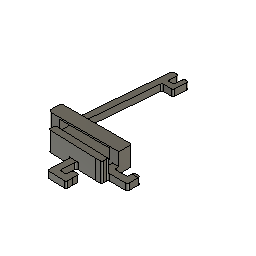
Keychain holder (Autodesk Fusion 360 design; units mm, degrees)
part number: 2026-04-03-17-33-08-056
Autodesk Fusion 360 part; units mm, degrees
note: some values were not read from the file. Chosen so that the rebuilt part matches the saved one: which bodies a step acts on.
sketch "Sketch1" plane through (0, 0, 0) normal (0, 0, 1) x (1, 0, 0)
  line L0 (0, 0) -> (0, 16.9)
  line L1 (0, 0) -> (-72.4203, 2.529)
  line L2 (0, 0) -> (75, 0) construction
  line L3 (0, 16.9) -> (-95, 16.9)
  line L4 (-100, 21.9) -> (-100, 34.4)
  line L5 (7.5, -10) -> (0, -10)
  line L6 (-75.0071, 0.0825) -> (-75.1109, -4.9108)
  line L7 (-89.5544, 39.1821) -> (-76.8804, 184.0471)
  line L8 (-79.7541, 36.9) -> (-9.7541, 36.9) construction
  line L9 (-74.3899, 186.3292) -> (-69.409, 186.3292)
  line L10 (-65.353, 170.3212) -> (-60.769, 170.3212)
  line L11 (-58.2785, 172.6033) -> (-57.3697, 182.9908)
  line L12 (-54.8792, 185.2729) -> (-52.7283, 185.2729)
  line L13 (-50.2378, 182.555) -> (-51.7942, 164.7646)
  line L14 (-54.2847, 162.4825) -> (-66.4762, 162.4825)
  line L15 (12.5, 10) -> (27.5, 10)
  line L16 (30, 12.5) -> (30, 17.5)
  line L17 (32.5, 20) -> (37.5, 20)
  line L18 (40, 17.5) -> (40, 2.5)
  line L19 (37.5, 0) -> (12.5, 0)
  line L20 (-30.1175, -11.4498) -> (-30.8155, -31.4376)
  line L21 (-28.4043, -34.0233) -> (-23.4057, -34.1979)
  line L22 (-10.9149, -34.6341) -> (-10.9149, -42.0453)
  line L23 (-13.5022, -44.5437) -> (-38.3982, -43.6743)
  line L24 (-40.8094, -41.0886) -> (-39.7626, -11.113)
  line L25 (-10.9149, -34.6341) -> (-10.6563, -27.2274)
  line L26 (-13.1548, -24.6402) -> (-18.1532, -24.6402)
  line L27 (-20.6517, -27.0513) -> (-20.8201, -31.7882)
  line L28 (-97.5, 36.9) -> (-92.0449, 36.9)
  line L29 (-77.0258, 36.9) -> (7.5, 36.9)
  line L30 (-66.9185, 183.6113) -> (-67.8435, 173.0391)
  line L31 (-68.9667, 160.2004) -> (-79.5163, 39.6179)
  line L32 (10, 34.4) -> (10, 12.5)
  line L33 (10, -2.5) -> (10, -7.5)
  line L34 (0, -10) -> (-27.5318, -9.0386)
  line L35 (-42.1739, -8.5273) -> (-72.6987, -7.4613)
  arc A0 (-74.3899, 186.3292) -> (-76.8804, 184.0471) centre (-74.3899, 183.8292) ccw
  arc A1 (-66.9185, 183.6113) -> (-69.409, 186.3292) centre (-69.409, 183.8292) ccw
  arc A2 (-50.2378, 182.555) -> (-52.7283, 185.2729) centre (-52.7283, 182.7729) ccw
  arc A3 (-54.8792, 185.2729) -> (-57.3697, 182.9908) centre (-54.8792, 182.7729) ccw
  arc A4 (-60.769, 170.3212) -> (-58.2785, 172.6033) centre (-60.769, 172.8212) ccw
  arc A5 (-67.8435, 173.0391) -> (-65.353, 170.3212) centre (-65.353, 172.8212) ccw
  arc A6 (-54.2847, 162.4825) -> (-51.7942, 164.7646) centre (-54.2847, 164.9825) ccw
  arc A7 (-66.4762, 162.4825) -> (-68.9667, 160.2004) centre (-66.4762, 159.9825) ccw
  arc A8 (-92.0449, 36.9) -> (-89.5544, 39.1821) centre (-92.0449, 39.4) ccw
  arc A9 (-79.5163, 39.6179) -> (-77.0258, 36.9) centre (-77.0258, 39.4) ccw
  arc A10 (10, 34.4) -> (7.5, 36.9) centre (7.5, 34.4) ccw
  arc A11 (10, 12.5) -> (12.5, 10) centre (12.5, 12.5) ccw
  arc A12 (27.5, 10) -> (30, 12.5) centre (27.5, 12.5) ccw
  arc A13 (32.5, 20) -> (30, 17.5) centre (32.5, 17.5) ccw
  arc A14 (40, 17.5) -> (37.5, 20) centre (37.5, 17.5) ccw
  arc A15 (37.5, 0) -> (40, 2.5) centre (37.5, 2.5) ccw
  arc A16 (12.5, 0) -> (10, -2.5) centre (12.5, -2.5) ccw
  arc A17 (7.5, -10) -> (10, -7.5) centre (7.5, -7.5) ccw
  arc A18 (-27.5318, -9.0386) -> (-30.1175, -11.4498) centre (-27.619, -11.537) ccw
  arc A19 (-30.8155, -31.4376) -> (-28.4043, -34.0233) centre (-28.317, -31.5249) ccw
  arc A20 (-23.4057, -34.1979) -> (-20.8201, -31.7882) centre (-23.3185, -31.6994) ccw
  arc A21 (-18.1532, -24.6402) -> (-20.6517, -27.0513) centre (-18.1532, -27.1402) ccw
  arc A22 (-10.6563, -27.2274) -> (-13.1548, -24.6402) centre (-13.1548, -27.1402) ccw
  arc A23 (-13.5022, -44.5437) -> (-10.9149, -42.0453) centre (-13.4149, -42.0453) ccw
  arc A24 (-40.8094, -41.0886) -> (-38.3982, -43.6743) centre (-38.3109, -41.1759) ccw
  arc A25 (-39.7626, -11.113) -> (-42.1739, -8.5273) centre (-42.2611, -11.0257) ccw
  arc A26 (-75.1109, -4.9108) -> (-72.6987, -7.4613) centre (-72.6115, -4.9628) ccw
  arc A27 (-72.4203, 2.529) -> (-75.0071, 0.0825) centre (-72.5076, 0.0305) ccw
  arc A28 (-97.5, 36.9) -> (-100, 34.4) centre (-97.5, 34.4) ccw
  arc A29 (-100, 21.9) -> (-95, 16.9) centre (-95, 21.9) ccw
  point P0 (-74.9543, 2.6175)
  point P1 (-100, 16.9)
  point P2 (-100, 36.9)
  point P3 (-89.7541, 36.9)
  point P4 (-76.6807, 186.3292)
  point P5 (30, 20)
  point P6 (40, 20)
  point P7 (-30.0303, -8.9513)
  point P8 (-30.9027, -33.9361)
  point P9 (-10.9149, -44.6341)
  point P10 (-40.8967, -43.5871)
  point P11 (-10.5659, -24.6402)
  point P12 (-20.5659, -24.6402)
  dimension "d9" = 16.9
  dimension "d10" = 178
  dimension "d11" = 75
  dimension "d12" = 100
  dimension "d13" = 20
  dimension "d14" = 178
  dimension "d15" = 85
  dimension "d16" = 150
  dimension "d17" = 10
  dimension "d19" = 10
  dimension "d20" = 25
  dimension "d21" = 20
  dimension "d22" = 10
  dimension "d23" = 30
  dimension "d24" = 10
  dimension "d25" = 10
  dimension "d26" = 2.5
  dimension "d27" = 5
  constraint coincident L0.start L1.start
  constraint vertical L0
  constraint horizontal L2
  constraint perpendicular L0 L3
  constraint perpendicular L3 L4
  constraint perpendicular L4 L28
  constraint perpendicular L2 L33
  constraint perpendicular L5 L33
  constraint horizontal L8
  constraint parallel L7 L30
  constraint horizontal L10
  constraint parallel L11 L30
  constraint horizontal L12
  constraint parallel L11 L13
  constraint parallel L12 L14
  constraint perpendicular L15 L32
  constraint perpendicular L15 L16
  constraint perpendicular L17 L32
  constraint perpendicular L2 L18
  constraint perpendicular L20 L34
  constraint perpendicular L20 L21
  constraint parallel L21 L23
  constraint perpendicular L24 L35
  constraint perpendicular L21 L25
  constraint perpendicular L22 L26
  constraint collinear L28 L29
  constraint collinear L30 L31
  constraint collinear L32 L33
  constraint collinear L34 L35
  constraint coincident P4 L7
  constraint coincident P4 L9
  constraint tangent L7 A0
  constraint tangent L9 A0
  constraint tangent L9 A1
  constraint tangent L30 A1
  constraint equal A0 A1
  constraint tangent L12 A2
  constraint tangent L13 A2
  constraint equal A0 A2
  constraint tangent L11 A3
  constraint tangent L12 A3
  constraint equal A0 A3
  constraint tangent L10 A4
  constraint tangent L11 A4
  constraint equal A0 A4
  constraint tangent L10 A5
  constraint tangent L30 A5
  constraint equal A0 A5
  constraint tangent L13 A6
  constraint tangent L14 A6
  constraint equal A0 A6
  constraint tangent L14 A7
  constraint tangent L31 A7
  constraint equal A0 A7
  constraint coincident P3 L7
  constraint coincident P3 L28
  constraint tangent L7 A8
  constraint tangent L28 A8
  constraint equal A0 A8
  constraint coincident L8.start L29
  constraint coincident L8.start L31
  constraint tangent L29 A9
  constraint tangent L31 A9
  constraint equal A0 A9
  constraint tangent L29 A10
  constraint tangent L32 A10
  constraint equal A0 A10
  constraint tangent L15 A11
  constraint tangent L32 A11
  constraint equal A0 A11
  constraint tangent L15 A12
  constraint tangent L16 A12
  constraint equal A0 A12
  constraint coincident P5 L16
  constraint coincident P5 L17
  constraint tangent L16 A13
  constraint tangent L17 A13
  constraint equal A0 A13
  constraint coincident P6 L17
  constraint coincident P6 L18
  constraint tangent L17 A14
  constraint tangent L18 A14
  constraint equal A0 A14
  constraint tangent L18 A15
  constraint tangent L19 A15
  constraint equal A0 A15
  constraint tangent L19 A16
  constraint tangent L33 A16
  constraint equal A0 A16
  constraint tangent L5 A17
  constraint tangent L33 A17
  constraint equal A0 A17
  constraint coincident P7 L20
  constraint coincident P7 L34
  constraint tangent L20 A18
  constraint tangent L34 A18
  constraint equal A0 A18
  constraint coincident P8 L20
  constraint coincident P8 L21
  constraint tangent L20 A19
  constraint tangent L21 A19
  constraint equal A0 A19
  constraint tangent L27 A20
  constraint tangent L21 A20
  constraint equal A0 A20
  constraint coincident P12 L26
  constraint coincident P12 L27
  constraint tangent L26 A21
  constraint tangent L27 A21
  constraint equal A0 A21
  constraint coincident P11 L25
  constraint coincident P11 L26
  constraint tangent L25 A22
  constraint tangent L26 A22
  constraint equal A0 A22
  constraint coincident P9 L22
  constraint coincident P9 L23
  constraint tangent L22 A23
  constraint tangent L23 A23
  constraint equal A0 A23
  constraint coincident P10 L23
  constraint coincident P10 L24
  constraint tangent L23 A24
  constraint tangent L24 A24
  constraint equal A0 A24
  constraint tangent L24 A25
  constraint tangent L35 A25
  constraint equal A0 A25
  constraint tangent L6 A26
  constraint tangent L35 A26
  constraint equal A0 A26
  constraint coincident P0 L1
  constraint coincident P0 L6
  constraint tangent L1 A27
  constraint tangent L6 A27
  constraint equal A0 A27
  constraint coincident P2 L4
  constraint coincident P2 L28
  constraint tangent L4 A28
  constraint tangent L28 A28
  constraint equal A0 A28
  constraint coincident P1 L3
  constraint coincident P1 L4
  constraint tangent L3 A29
  constraint tangent L4 A29
  measures "d9" distance of L0.start L0.end
  measures "d10" angle of L1 L2
  measures "d11" distance of L0.start P0
  measures "d12" distance of L0.end P1
  measures "d13" distance of P1 P2
  measures "d14" angle of L5 L34
  measures "d15" angle of L7 L8
  measures "d16" distance of P3 P4
  measures "d17" distance of P3 L8.start
  measures "d19" distance of P5 P6
  measures "d20" distance of P7 P8
  measures "d21" distance of P8 L22.start
  measures "d22" distance of L22.start P9
  measures "d23" distance of P9 P10
  measures "d24" distance of L22.start P11
  measures "d25" distance of P11 P12
  measures "d26" radius of A0
  measures "d27" radius of A29
extrude "Extrude1" add sketch "Sketch1" along normal blind 10 makes body 1
ref_plane "WorkPlane1" through (-47.5, 16.9, 5) normal (0, -1, 0) x (1, 0, 0)
ref_plane "WorkPlane2" through (-34.7629, 36.9, 5) normal (0, 1, 0) x (-1, 0, 0)
ref_plane "WorkPlane3" through (-13.7659, -9.5193, 5) normal (-0.034899, -0.999391, 0) x (0.999391, -0.034899, 0)
ref_plane "WorkPlane4" through (-36.2102, 1.2645, 5) normal (0.034899, 0.999391, 0) x (-0.999391, 0.034899, 0)
split "Split1" by plane through (-34.7629, 36.9, 5) normal (0, 1, 0) and through (-47.5, 16.9, 5) normal (0, -1, 0) and through (-13.7659, -9.5193, 5) normal (-0.034899, -0.999391, 0) and through (-36.2102, 1.2645, 5) normal (0.034899, 0.999391, 0) bodies 1 makes body 2 at (-37.1292, -27.8797, 0) makes body 3 at (34.1667, 20, 3.3333) makes body 4 at (-57.3419, 23.5667, 0) makes body 5 at (25.8333, 3.3333, 0) makes body 6 at (-78.4672, 127.8099, 0)
extrude "Extrude2" add 2 faces at (-57.3419, 23.5667, 10) (-38.1981, -1.9994, 10) along direction (0, 0, 1) blind 20 on bodies 1 4 bodies 1 4 2 5 6
sketch "Sketch2" plane through (0, 36.9, 0) normal (0, 1, 0) x (-1, 0, 0)
  line L0 (92.0449, 10) -> (92.0449, 0)
  line L1 (92.0449, 0) -> (97.5, 0)
  line L2 (97.5, 0) -> (97.5, 30)
  line L3 (97.5, 30) -> (-7.5, 30)
  line L4 (-7.5, 30) -> (-7.5, 0)
  line L5 (-7.5, 0) -> (77.0258, 0)
  line L6 (77.0258, 0) -> (77.0258, 10)
  line L7 (77.0258, 10) -> (92.0449, 10)
  line L8 (5.4, 27.5) -> (82.5, 27.5)
  line L9 (82.5, 27.5) -> (82.5, 11.5)
  line L10 (82.5, 11.5) -> (5.4, 11.5)
  line L11 (5.4, 11.5) -> (5.4, 27.5)
  dimension "d36" = 77.1
  dimension "d37" = 16
  dimension "d38" = 2.5
  dimension "d39" = 15
  constraint horizontal L8
  constraint vertical L9
  constraint horizontal L10
  constraint vertical L11
  measures "d36" distance of L8.start L8.end
  measures "d37" distance of L8.start L10.end
  measures "d38" distance of L3 L8
  measures "d39" distance of L2 L9
extrude "Extrude3" cut sketch "Sketch2" against normal blind 25 contours L8 L9 L10 L11 bodies 1
